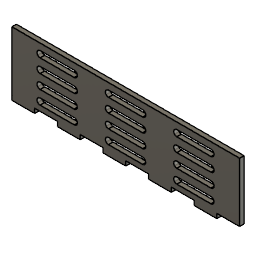
Lateral derecho e izquierdo (Autodesk Fusion 360 design; units mm, degrees)
Autodesk Fusion 360 part; units mm, degrees
sketch "Boceto1" plane through (0, 0, 0) normal (0, 0, 1) x (1, 0, 0)
  line L0 (-100, 26) -> (100, 26)
  line L1 (100, 26) -> (100, -26)
  line L2 (100, -26) -> (-100, -26)
  line L3 (-100, -26) -> (-100, 26)
  line L4 (-100, 26) -> (100, -26) construction
  line L5 (100, 26) -> (-100, -26) construction
  arc A0 (-45.1876, -21.2449) -> (-45.1876, -15.7551) centre (-45.1876, -18.5) ccw
  arc A1 (-75.1876, -15.7551) -> (-75.1876, -21.2449) centre (-75.1876, -18.5) ccw
  arc A2 (-75.1876, -3.7551) -> (-75.1876, -9.2449) centre (-75.1876, -6.5) ccw
  arc A3 (-75.1876, 20.2449) -> (-75.1876, 14.7551) centre (-75.1876, 17.5) ccw
  line L6 (-45.1876, -15.7551) -> (-75.1876, -15.7551)
  arc A4 (-45.1876, 2.7551) -> (-45.1876, 8.2449) centre (-45.1876, 5.5) ccw
  arc A5 (-45.1876, -9.2449) -> (-45.1876, -3.7551) centre (-45.1876, -6.5) ccw
  arc A6 (-45.1876, 14.7551) -> (-45.1876, 20.2449) centre (-45.1876, 17.5) ccw
  line L7 (-75.1876, -18.5) -> (-45.1876, -18.5) construction
  line L8 (-45.1876, 8.2449) -> (-75.1876, 8.2449)
  arc A7 (-75.1876, 8.2449) -> (-75.1876, 2.7551) centre (-75.1876, 5.5) ccw
  line L9 (-45.1876, 20.2449) -> (-75.1876, 20.2449)
  line L10 (-75.1876, -21.2449) -> (-45.1876, -21.2449)
  line L11 (-45.1876, -3.7551) -> (-75.1876, -3.7551)
  line L12 (-75.1876, 2.7551) -> (-45.1876, 2.7551)
  line L13 (-75.1876, 5.5) -> (-45.1876, 5.5) construction
  line L14 (-75.1876, -6.5) -> (-45.1876, -6.5) construction
  line L15 (-75.1876, 14.7551) -> (-45.1876, 14.7551)
  line L16 (-75.1876, -9.2449) -> (-45.1876, -9.2449)
  line L17 (-75.1876, 17.5) -> (-45.1876, 17.5) construction
  line L18 (-15.1318, 5.5) -> (14.8682, 5.5) construction
  arc A8 (14.8682, -9.2449) -> (14.8682, -3.7551) centre (14.8682, -6.5) ccw
  line L19 (14.8682, -3.7551) -> (-15.1318, -3.7551)
  arc A9 (14.8682, 14.7551) -> (14.8682, 20.2449) centre (14.8682, 17.5) ccw
  arc A10 (-15.1318, 8.2449) -> (-15.1318, 2.7551) centre (-15.1318, 5.5) ccw
  line L20 (14.8682, -15.7551) -> (-15.1318, -15.7551)
  arc A11 (-15.1318, -15.7551) -> (-15.1318, -21.2449) centre (-15.1318, -18.5) ccw
  arc A12 (-15.1318, -3.7551) -> (-15.1318, -9.2449) centre (-15.1318, -6.5) ccw
  line L21 (-15.1318, -21.2449) -> (14.8682, -21.2449)
  line L22 (-15.1318, -6.5) -> (14.8682, -6.5) construction
  line L23 (-15.1318, 17.5) -> (14.8682, 17.5) construction
  arc A13 (14.8682, -21.2449) -> (14.8682, -15.7551) centre (14.8682, -18.5) ccw
  arc A14 (14.8682, 2.7551) -> (14.8682, 8.2449) centre (14.8682, 5.5) ccw
  line L24 (-15.1318, -18.5) -> (14.8682, -18.5) construction
  arc A15 (-15.1318, 20.2449) -> (-15.1318, 14.7551) centre (-15.1318, 17.5) ccw
  line L25 (14.8682, 20.2449) -> (-15.1318, 20.2449)
  line L26 (-15.1318, 14.7551) -> (14.8682, 14.7551)
  line L27 (-15.1318, -9.2449) -> (14.8682, -9.2449)
  line L28 (14.8682, 8.2449) -> (-15.1318, 8.2449)
  line L29 (-15.1318, 2.7551) -> (14.8682, 2.7551)
  line L30 (74.8612, 20.2449) -> (44.8612, 20.2449)
  line L31 (74.8612, -3.7551) -> (44.8612, -3.7551)
  line L32 (44.8612, -9.2449) -> (74.8612, -9.2449)
  arc A16 (74.8612, -9.2449) -> (74.8612, -3.7551) centre (74.8612, -6.5) ccw
  line L33 (74.8612, -15.7551) -> (44.8612, -15.7551)
  arc A17 (74.8612, -21.2449) -> (74.8612, -15.7551) centre (74.8612, -18.5) ccw
  line L34 (44.8612, -6.5) -> (74.8612, -6.5) construction
  line L35 (44.8612, -21.2449) -> (74.8612, -21.2449)
  arc A18 (74.8612, 14.7551) -> (74.8612, 20.2449) centre (74.8612, 17.5) ccw
  line L36 (44.8612, 14.7551) -> (74.8612, 14.7551)
  line L37 (44.8612, -18.5) -> (74.8612, -18.5) construction
  line L38 (44.8612, 5.5) -> (74.8612, 5.5) construction
  arc A19 (44.8612, -3.7551) -> (44.8612, -9.2449) centre (44.8612, -6.5) ccw
  arc A20 (74.8612, 2.7551) -> (74.8612, 8.2449) centre (74.8612, 5.5) ccw
  line L39 (44.8612, 17.5) -> (74.8612, 17.5) construction
  line L40 (74.8612, 8.2449) -> (44.8612, 8.2449)
  line L41 (44.8612, 2.7551) -> (74.8612, 2.7551)
  arc A21 (44.8612, 20.2449) -> (44.8612, 14.7551) centre (44.8612, 17.5) ccw
  arc A22 (44.8612, 8.2449) -> (44.8612, 2.7551) centre (44.8612, 5.5) ccw
  arc A23 (44.8612, -15.7551) -> (44.8612, -21.2449) centre (44.8612, -18.5) ccw
  point P0 (59.993, 0)
  point P1 (59.993, 0)
  dimension "d1" = 200
  dimension "d2" = 52
  dimension "d3" = 30
  dimension "d4" = 30
  dimension "d5" = 30
  dimension "d6" = 12
  dimension "d7" = 12
  dimension "d8" = 30
  dimension "d9" = 12
  dimension "d10" = 30
  dimension "d11" = 30
  dimension "d12" = 30
  dimension "d13" = 12
  dimension "d14" = 12
  dimension "d15" = 30
  dimension "d16" = 12
  dimension "d17" = 30
  dimension "d18" = 30
  dimension "d19" = 30
  dimension "d20" = 12
  dimension "d21" = 12
  dimension "d22" = 30
  dimension "d23" = 12
  constraint horizontal L0
  constraint perpendicular L0 L1
  constraint parallel L0 L2
  constraint parallel L1 L3
  constraint coincident L4 origin
  constraint coincident L5 origin
  constraint tangent A6 L15
  constraint tangent A6 L9
  constraint parallel L9 L15
  constraint tangent A3 L9
  constraint tangent A3 L15
  constraint tangent A4 L12
  constraint tangent A4 L8
  constraint parallel L8 L12
  constraint tangent L8 A7
  constraint tangent A7 L12
  constraint tangent A5 L16
  constraint tangent A5 L11
  constraint parallel L11 L16
  constraint tangent A2 L11
  constraint tangent A2 L16
  constraint tangent A0 L10
  constraint tangent A0 L6
  constraint parallel L6 L10
  constraint tangent A1 L6
  constraint tangent A1 L10
  constraint tangent A9 L26
  constraint tangent A9 L25
  constraint parallel L25 L26
  constraint tangent A15 L25
  constraint tangent A15 L26
  constraint tangent A14 L29
  constraint tangent A14 L28
  constraint parallel L28 L29
  constraint tangent A10 L28
  constraint tangent A10 L29
  constraint tangent A8 L27
  constraint tangent A8 L19
  constraint parallel L19 L27
  constraint tangent L19 A12
  constraint tangent A12 L27
  constraint tangent L21 A13
  constraint tangent L20 A13
  constraint parallel L20 L21
  constraint tangent L20 A11
  constraint tangent A11 L21
  constraint coincident P1 P0
  constraint tangent A18 L36
  constraint tangent L30 A18
  constraint parallel L30 L36
  constraint tangent L30 A21
  constraint tangent L36 A21
  constraint tangent A20 L41
  constraint tangent A20 L40
  constraint parallel L40 L41
  constraint tangent L40 A22
  constraint tangent L41 A22
  constraint tangent L32 A16
  constraint tangent L31 A16
  constraint parallel L31 L32
  constraint tangent L31 A19
  constraint tangent L32 A19
  constraint tangent A17 L35
  constraint tangent L33 A17
  constraint parallel L33 L35
  constraint tangent L33 A23
  constraint tangent L35 A23
  measures "d1" distance of L1 L3
  measures "d2" distance of L0.start L2.end
  measures "d3" distance of A6.centre A3.centre
  measures "d4" distance of A7.centre A4.centre
  measures "d5" distance of A2.centre A5.centre
  measures "d6" distance of L13 L17
  measures "d7" distance of L13 L14
  measures "d8" distance of A0.centre A1.centre
  measures "d9" distance of L7 L14
  measures "d10" distance of L23.start A9.centre
  measures "d11" distance of L18.start L18.end
  measures "d12" distance of A8.centre A12.centre
  measures "d13" distance of L18 L23
  measures "d14" distance of L18 L22
  measures "d15" distance of A13.centre A11.centre
  measures "d16" distance of L22 L24
  measures "d17" distance of L39.start A18.centre
  measures "d18" distance of L38.start L38.end
  measures "d19" distance of A16.centre L34.start
  measures "d20" distance of L38 L39
  measures "d21" distance of L34 L38
  measures "d22" distance of A17.centre L37.start
  measures "d23" distance of L34 L37
extrude "Extruir1" add sketch "Boceto1" along normal blind 4
sketch "Boceto2" plane through (0, 0, 4) normal (0, 0, 1) x (1, 0, 0)
  line L0 (-45.1876, 14.7551) -> (-75.1876, 14.7551)
  arc A0 (-75.1876, 20.2449) -> (-75.1876, 14.7551) centre (-75.1876, 17.5) ccw
  line L1 (-75.1876, 20.2449) -> (-45.1876, 20.2449)
  arc A1 (-45.1876, 14.7551) -> (-45.1876, 20.2449) centre (-45.1876, 17.5) ccw
  line L2 (-45.1876, -9.2449) -> (-75.1876, -9.2449)
  arc A2 (-75.1876, -3.7551) -> (-75.1876, -9.2449) centre (-75.1876, -6.5) ccw
  line L3 (-75.1876, -3.7551) -> (-45.1876, -3.7551)
  arc A3 (-45.1876, -9.2449) -> (-45.1876, -3.7551) centre (-45.1876, -6.5) ccw
  line L4 (-100, -26) -> (100, -26)
  line L5 (100, -26) -> (100, 26)
  line L6 (100, 26) -> (-100, 26)
  line L7 (-100, 26) -> (-100, -26)
  arc A4 (44.8612, 20.2449) -> (44.8612, 14.7551) centre (44.8612, 17.5) ccw
  line L8 (44.8612, 20.2449) -> (74.8612, 20.2449)
  arc A5 (74.8612, 14.7551) -> (74.8612, 20.2449) centre (74.8612, 17.5) ccw
  line L9 (74.8612, 14.7551) -> (44.8612, 14.7551)
  line L10 (14.8682, -9.2449) -> (-15.1318, -9.2449)
  arc A6 (-15.1318, -3.7551) -> (-15.1318, -9.2449) centre (-15.1318, -6.5) ccw
  line L11 (-15.1318, -3.7551) -> (14.8682, -3.7551)
  arc A7 (14.8682, -9.2449) -> (14.8682, -3.7551) centre (14.8682, -6.5) ccw
  arc A8 (14.8682, -21.2449) -> (14.8682, -15.7551) centre (14.8682, -18.5) ccw
  line L12 (14.8682, -21.2449) -> (-15.1318, -21.2449)
  arc A9 (-15.1318, -15.7551) -> (-15.1318, -21.2449) centre (-15.1318, -18.5) ccw
  line L13 (-15.1318, -15.7551) -> (14.8682, -15.7551)
  line L14 (14.8682, 14.7551) -> (-15.1318, 14.7551)
  arc A10 (-15.1318, 20.2449) -> (-15.1318, 14.7551) centre (-15.1318, 17.5) ccw
  line L15 (-15.1318, 20.2449) -> (14.8682, 20.2449)
  arc A11 (14.8682, 14.7551) -> (14.8682, 20.2449) centre (14.8682, 17.5) ccw
  line L16 (-45.1876, -21.2449) -> (-75.1876, -21.2449)
  arc A12 (-75.1876, -15.7551) -> (-75.1876, -21.2449) centre (-75.1876, -18.5) ccw
  line L17 (-75.1876, -15.7551) -> (-45.1876, -15.7551)
  arc A13 (-45.1876, -21.2449) -> (-45.1876, -15.7551) centre (-45.1876, -18.5) ccw
  arc A14 (44.8612, -15.7551) -> (44.8612, -21.2449) centre (44.8612, -18.5) ccw
  line L18 (44.8612, -15.7551) -> (74.8612, -15.7551)
  arc A15 (74.8612, -21.2449) -> (74.8612, -15.7551) centre (74.8612, -18.5) ccw
  line L19 (74.8612, -21.2449) -> (44.8612, -21.2449)
  line L20 (-45.1876, 2.7551) -> (-75.1876, 2.7551)
  arc A16 (-75.1876, 8.2449) -> (-75.1876, 2.7551) centre (-75.1876, 5.5) ccw
  line L21 (-75.1876, 8.2449) -> (-45.1876, 8.2449)
  arc A17 (-45.1876, 2.7551) -> (-45.1876, 8.2449) centre (-45.1876, 5.5) ccw
  arc A18 (44.8612, 8.2449) -> (44.8612, 2.7551) centre (44.8612, 5.5) ccw
  line L22 (44.8612, 8.2449) -> (74.8612, 8.2449)
  arc A19 (74.8612, 2.7551) -> (74.8612, 8.2449) centre (74.8612, 5.5) ccw
  line L23 (74.8612, 2.7551) -> (44.8612, 2.7551)
  line L24 (14.8682, 2.7551) -> (-15.1318, 2.7551)
  arc A20 (-15.1318, 8.2449) -> (-15.1318, 2.7551) centre (-15.1318, 5.5) ccw
  line L25 (-15.1318, 8.2449) -> (14.8682, 8.2449)
  arc A21 (14.8682, 2.7551) -> (14.8682, 8.2449) centre (14.8682, 5.5) ccw
  arc A22 (44.8612, -3.7551) -> (44.8612, -9.2449) centre (44.8612, -6.5) ccw
  line L26 (44.8612, -3.7551) -> (74.8612, -3.7551)
  arc A23 (74.8612, -9.2449) -> (74.8612, -3.7551) centre (74.8612, -6.5) ccw
  line L27 (74.8612, -9.2449) -> (44.8612, -9.2449)
  line L28 (80, -26) -> (80, -30)
  line L29 (80, -30) -> (60, -30)
  line L30 (60, -30) -> (60, -26)
  line L31 (40, -26) -> (40, -30)
  line L32 (40, -30) -> (20, -30)
  line L33 (20, -30) -> (20, -26)
  line L34 (0, -26) -> (0, -30)
  line L35 (0, -30) -> (-20, -30)
  line L36 (-20, -30) -> (-20, -26)
  line L37 (-40, -26) -> (-40, -30)
  line L38 (-40, -30) -> (-60, -30)
  line L39 (-60, -30) -> (-60, -26)
  line L40 (-80, -26) -> (-80, -30)
  line L41 (-80, -30) -> (-100, -30)
  line L42 (-100, -30) -> (-100, -26)
  line L43 (80, -26) -> (60, -26)
  line L44 (40, -26) -> (20, -26)
  line L45 (0, -26) -> (-20, -26)
  line L46 (-40, -26) -> (-60, -26)
  line L47 (-80, -26) -> (-100, -26)
  dimension "d36" = 20
  dimension "d37" = 20
  dimension "d38" = 20
  dimension "d39" = 20
  dimension "d40" = 20
  dimension "d41" = 20
  dimension "d42" = 20
  dimension "d43" = 20
  dimension "d44" = 20
  constraint coincident L4 L28.start
  constraint coincident L4 L30.end
  constraint coincident L4 L31.start
  constraint coincident L4 L33.end
  constraint midpoint L4 L34.start
  constraint coincident L4 L36.end
  constraint coincident L4 L37.start
  constraint coincident L4 L39.end
  constraint coincident L4 L40.start
  constraint perpendicular L4 L28
  constraint perpendicular L28 L29
  constraint perpendicular L4 L31
  constraint perpendicular L31 L32
  constraint perpendicular L4 L33
  constraint perpendicular L4 L34
  constraint perpendicular L4 L37
  constraint perpendicular L37 L38
  constraint perpendicular L4 L40
  constraint perpendicular L40 L41
  constraint coincident L4.start L7.end
  measures "d36" distance of L28 L30
  measures "d37" distance of L30 L31
  measures "d38" distance of L31.end L32.end
  measures "d39" distance of L33 L34
  measures "d40" distance of L34 L36
  measures "d41" distance of L36 L37
  measures "d42" distance of L37 L39
  measures "d43" distance of L39 L40
  measures "d44" distance of L40 L42
extrude "Extruir2" add sketch "Boceto2" against normal blind 4 contours L4 L40 L41 L42 L47 | L4 L37 L38 L39 L46 | L4 L34 L35 L36 L45 | L4 L28 L29 L30 L43 | L4 L31 L32 L33 L44
